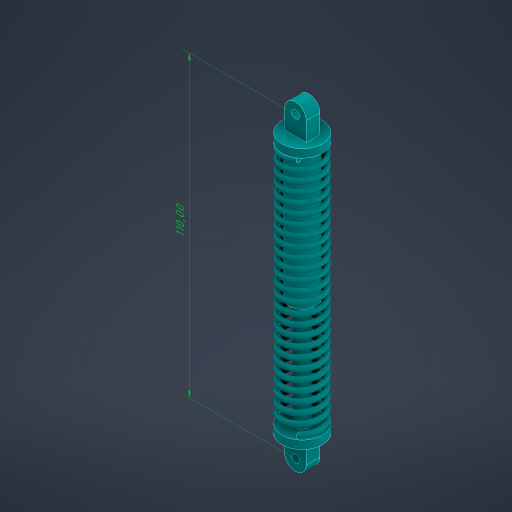
# Autodesk Inventor part: shock_absorber
Saved by Autodesk Inventor 2024 (Build 280153000, 153)
## iProperties
Created: 2023-04-13
Part Number: shock_absorber
Material: Типовые
Document SubType Name: Modeling
Designer: user
Density: 1 g/cm^3
Appearance: По умолчанию
Author: user
Autodesk Inventor part; units mm, degrees
ref_plane "YZ Plane" through (0, 0, 0) normal (1, 0, 0) x (0, 1, 0)
ref_plane "XZ Plane" through (0, 0, 0) normal (0, 1, 0) x (-1, 0, 0)
ref_plane "XY Plane" through (0, 0, 0) normal (0, 0, 1) x (1, 0, 0)
sketch "Эскиз1" plane through (0, 0, 0) normal (0, 0, 1) x (1, 0, 0)
  circle A0 centre (0, 0) radius 1.5
  arc A1 (-4, 0) -> (4, 0) centre (0, 0) ccw
  line L0 (-4, 0) -> (-4, 10)
  line L1 (4, 0) -> (4, 10)
  line L2 (-4, 10) -> (4, 10)
  circle A2 centre (0, 110) radius 1.5
  arc A3 (4, 110) -> (-4, 110) centre (0, 110) ccw
  line L3 (-4, 110) -> (-4, 100)
  line L4 (4, 110) -> (4, 100)
  line L5 (4, 100) -> (-4, 100)
  point P0 (0, 100)
  point P1 (0, 10)
  dimension "d0" = 3
  dimension "d1" = 8
  dimension "d2" = 10
  dimension "d8" = 110
  constraints: 12 end point, 4 centre point, 4 point on circle, 4 tangent, 4 vertical, 3 coincident, 2 equal radius, 2 midpoint, 2 vertical alignment, 1 collinear, 1 horizontal, 1 perpendicular
  measures "d0" diameter of A0
  measures "d1" diameter of A1
  measures "d2" vertical distance of point (0, 0) L0.end
  measures "d8" distance of point (0, 0) A2.centre
extrude "Выдавливание1" add sketch "Эскиз1" along normal blind 5
sketch "Эскиз2" plane through (-4, 10, 0) normal (0, 1, 0) x (1, 0, 0)
  circle A0 centre (4, -2.5) radius 7.5
  line L0 (8, 0) -> (0, 0) projected
  line L1 (8, 0) -> (8, -5) projected
  point P0 (4, 0)
  point P1 (4, 0)
  point P2 (8, -2.5)
  dimension "d5" = 15
  constraints: 2 midpoint, 1 centre point, 1 horizontal alignment, 1 vertical alignment
  measures "d5" diameter of A0
extrude "Выдавливание2" add sketch "Эскиз2" against normal blind 3
sketch "Эскиз3" plane through (-4, 100, 0) normal (0, -1, 0) x (1, 0, 0)
  circle A0 centre (4, 2.5) radius 7.5
  circle A1 centre (4, 2.5) radius 7.5 projected
  line L0 (0, 5) -> (8, 5) projected
  line L1 (8, 0) -> (8, 5) projected
  point P0 (4, 0)
  point P1 (4, 5)
  point P2 (8, 2.5)
  constraints: 2 midpoint, 1 centre point, 1 concentric, 1 horizontal alignment, 1 vertical alignment
extrude "Выдавливание3" add sketch "Эскиз3" against normal blind 3
sketch "Эскиз4" plane through (0, 100, 2.5) normal (0, -1, 0) x (1, 0, 0)
  circle A0 centre (0, 0) radius 5
  line L0 (4, -2.5) -> (4, 2.5) projected
  line L1 (-4, -2.5) -> (4, -2.5) projected
  point P0 (0, -2.5)
  point P1 (4, 0)
  point P2 (0, -2.5)
  dimension "d11" = 10
  constraints: 2 midpoint, 1 centre point, 1 horizontal alignment, 1 vertical alignment
  measures "d11" diameter of A0
extrude "Выдавливание4" add sketch "Эскиз4" along normal blind 50
sketch "Эскиз5" plane through (0, 50, 2.5) normal (0, -1, 0) x (1, 0, 0)
  circle A0 centre (0, 0) radius 2.5
  line L0 (4, -2.5) -> (4, 2.5) projected
  line L1 (-4, -2.5) -> (4, -2.5) projected
  point P0 (0, -2.5)
  point P1 (4, 0)
  point P2 (0, -2.5)
  dimension "d14" = 5
  constraints: 2 midpoint, 1 centre point, 1 horizontal alignment, 1 vertical alignment
  measures "d14" diameter of A0
extrude "Выдавливание5" add sketch "Эскиз5" along normal up to surface (40 mm away)
sketch "Эскиз7" plane through (4, 0, 5) normal (1, 0, 0) x (0, 0, -1)
  circle A0 centre (-2.8069, 11) radius 1
  point P0 (5, 0)
  dimension "d17" = 11
  dimension "d18" = 2
  constraints: 1 centre point
  measures "d17" vertical distance of A0.centre point (5, 0)
  measures "d18" diameter of A0
coil "Пружина1" sketch "Эскиз7" operation add axis through (0, 100, 2.5) along (0, 1, 0) pitch 3.52 turns 25 hand right
